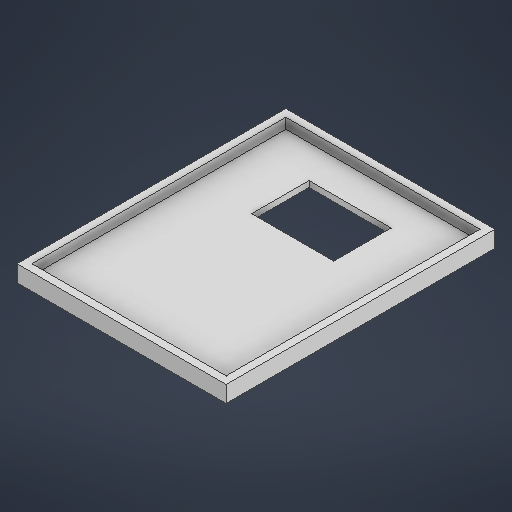
# Autodesk Inventor part: Tampa
Saved by Autodesk Inventor 2025 (Build 290162010, 162A)
## iProperties
Created: 2024-07-29
Part Number: Tampa
Material: Generic
Document SubType Name: Modeling
Designer: GabrielDBN
Density: 1 g/cm^3
Appearance: Default
Author: GabrielDBN
Autodesk Inventor part; units mm, degrees
ref_plane "YZ Plane" through (0, 0, 0) normal (1, 0, 0) x (0, 1, 0)
ref_plane "XZ Plane" through (0, 0, 0) normal (0, 1, 0) x (-1, 0, 0)
ref_plane "XY Plane" through (0, 0, 0) normal (0, 0, 1) x (1, 0, 0)
sketch "Sketch1" plane through (0, 0, 0) normal (0, 1, 0) x (-1, 0, 0)
  line L0 (32.6378, 42.945) -> (-32.3622, 42.945)
  line L1 (32.6378, 42.945) -> (32.6378, -42.055)
  line L2 (32.6378, -42.055) -> (-32.3622, -42.055)
  line L3 (-32.3622, -42.055) -> (-32.3622, 42.945)
  line L4 (-34.8622, 45.445) -> (35.1378, 45.445)
  line L5 (35.1378, -44.555) -> (-34.8622, -44.555)
  line L6 (35.1378, -44.555) -> (35.1378, 45.445)
  line L7 (-34.8622, -44.555) -> (-34.8622, 45.445)
  point P0 (0, 0)
  dimension "d0" = 65
  dimension "d1" = 85
  dimension "d6" = 70
  dimension "d7" = 90
  constraints: 16 end point, 4 horizontal, 2 vertical, 1 parallel, 1 perpendicular
  measures "d0" distance of L0.start L0.end
  measures "d1" distance of L0.start L1.end
  measures "d6" distance of L4.start L4.end
  measures "d7" distance of L5.start L4.end
extrude "Extrusion1" add sketch "Sketch1" along normal blind 2 contours L1 L2 L3 L0
extrude "Extrusion2" add sketch "Sketch1" along normal blind 5.5
sketch "Sketch2" plane through (0, 2, 0) normal (0, 1, 0) x (1, 0, 0)
  line L0 (32.3622, 42.055) -> (-32.6378, 42.055) projected
  line L1 (13.6122, 31.055) -> (13.6122, 11.855)
  line L2 (13.6122, 11.855) -> (-13.8878, 11.855)
  line L3 (-13.8878, 11.855) -> (-13.8878, 31.055)
  line L4 (-13.8878, 31.055) -> (13.6122, 31.055)
  point P0 (0, 0)
  dimension "d15" = 19.2
  dimension "d16" = 27.5
  constraints: 8 end point, 2 perpendicular, 1 horizontal, 1 vertical
  measures "d15" distance of L1.start L1.end
  measures "d16" distance of L1.end L2.end
extrude "Extrusion3" cut sketch "Sketch2" against normal blind 5
body "Solid1"
